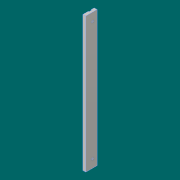
# Autodesk Inventor part: mppcMountClamp
Saved by Autodesk Inventor 2016 (Build 200138000, 138)
## iProperties
Created: 2016-02-18
Part Number: mppcMountClamp
Material: Aluminum 6061
Document SubType Name: Modeling
Designer: Sawaiz
Density: 2.7 g/cm^3
Appearance: Aluminum - Flat
Author: Sawaiz
Autodesk Inventor part; units mm, degrees
ref_plane "YZ Plane" through (0, 0, 0) normal (1, 0, 0) x (0, 1, 0)
ref_plane "XZ Plane" through (0, 0, 0) normal (0, 1, 0) x (-1, 0, 0)
ref_plane "XY Plane" through (0, 0, 0) normal (0, 0, 1) x (1, 0, 0)
sketch "Sketch1" plane through (0, 0, 0) normal (0, 1, 0) x (-1, 0, 0)
  line L0 (-5.7, -114) -> (5.7, -114)
  line L1 (5.7, -114) -> (5.7, 114)
  line L2 (5.7, 114) -> (-5.7, 114)
  line L3 (-5.7, 114) -> (-5.7, -114)
  line L4 (-5.7, -114) -> (5.7, 114) construction
  line L5 (5.7, -114) -> (-5.7, 114) construction
  line L6 (-12.5, -150) -> (12.5, -150)
  line L7 (12.5, -150) -> (12.5, 150)
  line L8 (12.5, 150) -> (-12.5, 150)
  line L9 (-12.5, 150) -> (-12.5, -150)
  line L10 (-12.5, -150) -> (12.5, 150) construction
  line L11 (12.5, -150) -> (-12.5, 150) construction
  point P0 (0, 0)
  dimension "d0" = 11.4
  dimension "d1" = 228
  dimension "d2" = 300
  dimension "d3" = 25
  constraints: 24 end point, 4 midpoint, 4 parallel, 2 horizontal, 2 perpendicular
  measures "d0" distance of L1.end L2.end
  measures "d1" distance between parallel lines of L0 L2
  measures "d2" distance of L6.end L7.end
  measures "d3" distance of L7.end L8.end
extrude "Extrusion1" add sketch "Sketch1" along normal blind 6.35
sketch "Sketch2" plane through (0, 6.35, 0) normal (0, 1, 0) x (1, 0, 0)
  line L0 (5.7, 114) -> (5.7, -114) projected
  line L1 (5.7, -114) -> (-5.7, -114) projected
  line L2 (-5.7, -114) -> (-5.7, 114) projected
  line L3 (-5.7, 114) -> (5.7, 114) projected
  line L4 (12.5, 150) -> (-12.5, 150) projected
  line L5 (-12.5, 150) -> (-12.5, -150) projected
  line L6 (-12.5, -150) -> (12.5, -150) projected
  line L7 (12.5, -150) -> (12.5, 150) projected
  point P0 (0, 0)
extrude "Extrusion2" add sketch "Sketch2" against normal blind 3.175 contours L0 L1 L2 L3
sketch "Sketch3" plane through (0, 0, 0) normal (0, -1, 0) x (1, 0, 0)
  line L0 (5.7, 114) -> (5.7, -114) projected
  line L1 (5.7, -114) -> (-5.7, -114) projected
  line L2 (-5.7, -114) -> (-5.7, 114) projected
  line L3 (-5.7, 114) -> (5.7, 114) projected
  line L4 (12.5, -150) -> (-12.5, -150) projected
  line L5 (12.5, 150) -> (12.5, -150) projected
  line L6 (-12.5, 150) -> (12.5, 150) projected
  line L7 (-12.5, -150) -> (-12.5, 150) projected
  point P0 (0, 0)
  point P1 (-2.5, -132)
  dimension "d8" = 18
  dimension "d36" = 10
  measures "d8" distance from line of L4 point (-2.5, -132)
  measures "d36" distance from line of L7 point (-2.5, -132)
hole "Hole1" at (-2.5, 0, -132) direction (0, 1, 0) diameter 4.134 depth 14.2 tip angle 118 thread size "M5x0.8" class "6H" standard "ANSI Metric M Profile"
sketch "Sketch4" plane through (0, 0, 0) normal (0, -1, 0) x (1, 0, 0)
  circle A0 centre (-2.5, -132) radius 2.067 projected
  line L0 (5.7, 114) -> (5.7, -114) projected
  line L1 (5.7, -114) -> (-5.7, -114) projected
  line L2 (-5.7, -114) -> (-5.7, 114) projected
  line L3 (-5.7, 114) -> (5.7, 114) projected
  line L4 (12.5, -150) -> (-12.5, -150) projected
  line L5 (12.5, 150) -> (12.5, -150) projected
  line L6 (-12.5, 150) -> (12.5, 150) projected
  line L7 (-12.5, -150) -> (-12.5, 150) projected
  line L8 (-5.675, -150) -> (0.675, -150)
  line L9 (0.675, -150) -> (0.675, -124.6)
  line L10 (0.675, -124.6) -> (-5.675, -124.6)
  line L11 (-5.675, -124.6) -> (-5.675, -150)
  line L12 (-2.5, -124.6) -> (-2.5, -132) construction
  point P0 (0, 0)
  dimension "d17" = 6.35
  dimension "d18" = 25.4
  constraints: 10 end point, 2 parallel, 1 horizontal, 1 midpoint, 1 perpendicular, 1 point on line, 1 vertical
  measures "d17" distance of L9.end L10.end
  measures "d18" distance between parallel lines of L4 L10
extrude "Extrusion3" cut sketch "Sketch4" against normal blind 1.5875 contours L4 L11 L10 L9
fillet "Fillet1" radius 3.175 2 edges at (-5.675, 0.7937, -124.6) (0.675, 0.7937, -124.6)
mirror "Mirror1" about plane through (0, 0, 0) normal (0, 0, 1) of "Hole1", "Extrusion3", "Fillet1"
sketch "Sketch7" plane through (0, 0, 0) normal (0, -1, 0) x (1, 0, 0)
  line L0 (5.7, 114) -> (5.7, -114) projected
  line L1 (5.7, -114) -> (-5.7, -114) projected
  line L2 (-5.7, -114) -> (-5.7, 114) projected
  line L3 (-5.7, 114) -> (5.7, 114) projected
  line L4 (0.675, 150) -> (0.675, 127.775) projected
  arc A0 (-5.675, 127.775) -> (0.675, 127.775) centre (-2.5, 127.775) ccw projected
  line L5 (-5.675, 127.775) -> (-5.675, 150) projected
  line L6 (-12.5, 150) -> (-5.675, 150) projected
  line L7 (-12.5, -150) -> (-12.5, 150) projected
  line L8 (-5.675, -150) -> (-12.5, -150) projected
  line L9 (-5.675, -150) -> (-5.675, -127.775) projected
  arc A1 (0.675, -127.775) -> (-5.675, -127.775) centre (-2.5, -127.775) ccw projected
  line L10 (0.675, -127.775) -> (0.675, -150) projected
  line L11 (12.5, -150) -> (0.675, -150) projected
  line L12 (12.5, 150) -> (12.5, -150) projected
  line L13 (0.675, 150) -> (12.5, 150) projected
  line L14 (-5.7, 114) -> (5.7, 114) projected
  arc A2 (5.7, 114) -> (-5.7, 114) centre (0, 114) ccw
  line L15 (-5.7, -114) -> (-5.7, 114) projected
  arc A3 (-5.7, -114) -> (5.7, -114) centre (0, -114) ccw
  line L16 (5.7, 114) -> (5.7, -114) projected
  point P0 (0, 0)
  constraints: 4 point on circle, 2 centre point, 2 tangent
extrude "Extrusion5" cut sketch "Sketch7" against normal up to surface (3.175 mm away) contours L3 A2 | A3 L1
equation "\"d0\" = 2 * rubberizedCoating + ScintillatorWidth + 2 * silveringThickness"
equation "\"d1\" = 20 * d0"
equation "\"d4\" = mppcMountDepth"
equation "\"d6\" = 0.5 * mppcMountDepth"
equation "\"silveringThickness\" = 0.2"
equation "\"rubberizedCoating\" = 0.5"
equation "\"mppcMountDepth\" = 6.35"
equation "\"OpticalFiberDiameter\" = 1"
equation "\"OpticalFiberClearence\" = 0.1"
equation "\"ScintillatorEdgeClearence\" = 3"
equation "\"ShallowTrackDepth\" = 1.2"
equation "\"DeepTrackDepth\" = 5.6"
equation "\"FiberEdgeOffsett\" = 5"
equation "\"LoopLargeTrackRatio\" = 1.1"
equation "\"FiberSensorClerence\" = 0.5"
equation "\"MountingScrewOffsett\" = 9"
equation "\"ScintillatorWidth\" = 10"
body "Solid1"
